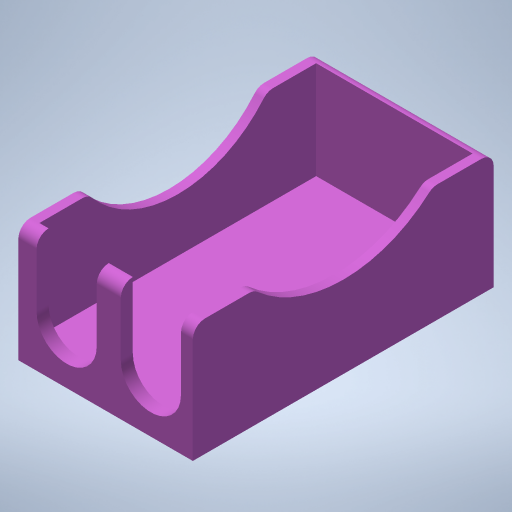
# Autodesk Inventor part: CASE batería
Saved by Autodesk Inventor 2024 (Build 280153000, 153)
## iProperties
Created: 2024-06-15
Part Number: CASE batería
Material: Genérico
Document SubType Name: Modeling
Designer: Valeria
Density: 1 g/cm^3
Appearance: Por defecto
Author: Valeria
Autodesk Inventor part; units mm, degrees
ref_plane "YZ Plane" through (0, 0, 0) normal (1, 0, 0) x (0, 1, 0)
ref_plane "XZ Plane" through (0, 0, 0) normal (0, 1, 0) x (-1, 0, 0)
ref_plane "XY Plane" through (0, 0, 0) normal (0, 0, 1) x (1, 0, 0)
sketch "Boceto1" plane through (0, 0, 0) normal (0, 1, 0) x (-1, 0, 0)
  line L0 (-13, -23) -> (13, -23)
  line L1 (13, -23) -> (13, 23)
  line L2 (13, 23) -> (-13, 23)
  line L3 (-13, 23) -> (-13, -23)
  line L4 (-13, -23) -> (13, 23) construction
  line L5 (13, -23) -> (-13, 23) construction
  line L6 (-14.5, -25) -> (14.5, -25)
  line L7 (14.5, -25) -> (14.5, 25)
  line L8 (14.5, 25) -> (-14.5, 25)
  line L9 (-14.5, 25) -> (-14.5, -25)
  line L10 (-14.5, -25) -> (14.5, 25) construction
  line L11 (14.5, -25) -> (-14.5, 25) construction
  point P0 (0, 0)
  dimension "d0" = 46
  dimension "d1" = 26
  dimension "d2" = 2
  dimension "d3" = 1.5
  constraints: 24 end point, 4 midpoint, 4 parallel, 2 horizontal, 2 perpendicular
  measures "d0" distance of L0.end L1.end
  measures "d1" distance of L1.end L2.end
  measures "d2" distance between parallel lines of L8 L2
  measures "d3" distance between parallel lines of L7 L1
extrude "Extrusión1" add sketch "Boceto1" along normal blind 19.5 contours L3 L2 L1 L0 | L9 L8 L7 L6
sketch "Boceto2" plane through (0, 19.5, 0) normal (0, 1, 0) x (1, 0, 0)
  line L0 (-13, -23) -> (13, -23) projected
  line L1 (13, -23) -> (13, 23) projected
  line L2 (13, 23) -> (-13, 23) projected
  line L3 (-13, 23) -> (-13, -23) projected
  point P0 (0, 0)
extrude "Extrusión2" cut sketch "Boceto2" against normal blind 16.25
sketch "Boceto3" plane through (-14.5, 0, 25) normal (0, 0, 1) x (1, 0, 0)
  line L0 (29, 19.5) -> (0, 19.5) projected
  line L1 (13.0274, 19.5) -> (13.0274, 8.5)
  line L2 (17.0274, 19.5) -> (17.0274, 8.5)
  line L3 (3.0274, 19.5) -> (3.0274, 8.5)
  line L4 (27.0274, 19.5) -> (27.0274, 8.5)
  arc A0 (3.0274, 8.5) -> (13.0274, 8.5) centre (8.0274, 8.5) ccw
  arc A1 (17.0274, 8.5) -> (27.0274, 8.5) centre (22.0274, 8.5) ccw
  point P0 (14.5, 0)
  dimension "d8" = 11
  dimension "d10" = 10
  dimension "d11" = 10
  dimension "d12" = 4
  dimension "d13" = 11
  dimension "d14" = 11
  dimension "d15" = 11
  constraints: 8 end point, 4 point on circle, 4 point on line, 4 vertical, 2 centre point
  measures "d8" distance of L3.start L3.end
  measures "d10" distance between parallel lines of L4 L2
  measures "d11" distance between parallel lines of L1 L3
  measures "d12" distance between parallel lines of L2 L1
  measures "d13" distance of L4.start L4.end
  measures "d14" distance of L2.start L2.end
  measures "d15" distance of L1.start L1.end
extrude "Extrusión3" cut sketch "Boceto3" against normal blind 17
sketch "Boceto4" plane through (-14.5, 0, -25) normal (-1, 0, 0) x (0, 0, 1)
  line L0 (48, 19.5) -> (2, 19.5) projected
  arc A0 (10.16, 19.5) -> (39.84, 19.5) centre (25, 30.7495) ccw
  line L1 (0, 0) -> (0, 19.5) projected
  line L2 (50, 0) -> (50, 19.5) projected
  point P0 (25, 0)
  dimension "d18" = 10.16
  dimension "d19" = 10.16
  constraints: 2 point on circle, 2 point on line, 1 centre point
  measures "d18" distance from line of L1 A0.start
  measures "d19" distance from line of L2 A0.end
extrude "Extrusión4" cut sketch "Boceto4" against normal blind 17
sketch "Boceto5" plane through (14.5, 0, 25) normal (1, 0, 0) x (0, 0, -1)
  line L0 (48, 19.5) -> (2, 19.5) projected
  arc A0 (10.16, 19.5) -> (39.84, 19.5) centre (25, 35.1546) ccw
  line L1 (50, 0) -> (50, 19.5) projected
  line L2 (0, 0) -> (0, 19.5) projected
  point P0 (25, 0)
  dimension "d22" = 10.16
  dimension "d23" = 10.16
  constraints: 2 point on circle, 2 point on line, 1 centre point
  measures "d22" distance from line of L1 A0.end
  measures "d23" distance from line of L2 A0.start
extrude "Extrusión5" cut sketch "Boceto5" against normal blind 17
fillet "Empalme1" radius 2 8 edges at (13.75, 19.5, -14.84) (13.75, 19.5, 14.84) (13.5137, 19.5, 25) (-13.75, 19.5, -14.84) (-13.75, 19.5, 14.84) (-12.9863, 19.5, 25) (0.5274, 19.5, 25) (0, 19.5, -25)
